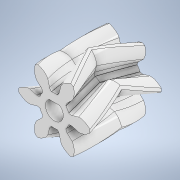
# Autodesk Inventor part: DoubleHelicalDriveGear
Saved by Autodesk Inventor 2020.2 (Build 242310000, 310)
## iProperties
Created: 2019-09-23
Part Number: DoubleHelicalDriveGear
Material: Generic
Document SubType Name: Modeling
Designer: Eric
Density: 1 g/cm^3
Appearance: White
ReferenceDiameter: 15.000 mm
Teeth: 6.000 ul
TipDiameter: 20.000 mm
Author: Eric
Autodesk Inventor part; units mm, degrees
ref_plane "YZ Plane" through (0, 0, 0) normal (1, 0, 0) x (0, 1, 0)
ref_plane "XZ Plane" through (0, 0, 0) normal (0, 1, 0) x (-1, 0, 0)
ref_plane "XY Plane" through (0, 0, 0) normal (0, 0, 1) x (1, 0, 0)
sketch "Sketch1" plane through (0, 0, 0) normal (0, 0, 1) x (1, 0, 0)
  circle A0 centre (0, 0) radius 7.0477
  circle A1 centre (0, 0) radius 7.5
  circle A2 centre (0, 0) radius 10
  circle A3 centre (0, 0) radius 4.375
  line L0 (-14, 0) -> (14, 0) projected
  line L1 (0, 0) -> (6.8335, 1.7241)
  line L2 (7.2444, 1.9411) -> (0, 0)
  line L3 (7.2444, 1.9411) -> (0, 0)
  circle A4 centre (0, 0) radius 7.0477
  dimension "BaseDiameter" = 14.0954
  dimension "RootDiameter" = 8.75
  dimension "ReferenceDiameter" = 15
  dimension "TipDiameter" = 20
  dimension "d26" = 15
  dimension "d30" = 15
  dimension "d48" = 0.7398
  constraints: 6 end point, 4 coincident, 3 centre point, 2 horizontal, 2 point on circle, 1 line through centre, 1 point on line, 20 other
  measures "ReferenceDiameter" diameter of A1
  measures "TipDiameter" diameter of A2
  measures "d26" angle of L0 L2
  measures "d30" angle of L0 L3
  measures "d48" distance from line of L0 point (4.312, 0.74)
extrude "Extrusion3" add sketch "Sketch1" along normal blind 10
sketch "Sketch3" plane through (0, 0, 0) normal (0, 0, 1) x (1, 0, 0)
  circle A0 centre (0, 0) radius 10 projected
  circle A1 centre (0, 0) radius 4.375 projected
  line L0 (0, 0) -> (6.8335, 1.7241) projected
  spline S0 degree 3 poles (4.312, 0.7398) (4.6304, 1.2842) (5.5617, 1.5626) (6.6593, 1.13) (7.1921, 0.9201) (7.7578, 0.5477) (8.2812, 0) knots -0.027536 -0.027536 -0.027536 -0.027536 0.566373 0.566373 0.566373 0.854705 0.854705 0.854705 0.854705 projected
  spline S1 degree 3 poles (6.8335, 1.7241) (6.9431, 1.7526) (7.0448, 1.8131) (7.1455, 1.8759) (7.8344, 2.3054) (8.4145, 3.1058) (8.8099, 4.097) (8.9564, 4.4642) (9.0767, 4.8606) (9.1662, 5.2815) knots 1 1 1 1 1.048198 1.048198 1.048198 1.377882 1.377882 1.377882 1.5 1.5 1.5 1.5 projected
  circle A2 centre (0, 0) radius 10 projected
  circle A3 centre (0, 0) radius 4.275
  line L1 (-0.0245, 0.097) -> (6.8087, 1.821)
  line L2 (-14, 0) -> (14, 0) projected
  arc A4 (4.217, 0.7953) -> (4.2088, 0.7493) centre (4.2755, 0.7611) ccw
  line L3 (-0.0245, -0.097) -> (6.8087, -1.821)
  spline S2 degree 3 poles (4.312, -0.7398) (4.6304, -1.2842) (5.5617, -1.5626) (6.6593, -1.13) (7.1921, -0.9201) (7.7578, -0.5477) (8.2812, 0) knots -0.027536 -0.027536 -0.027536 -0.027536 0.566373 0.566373 0.566373 0.854705 0.854705 0.854705 0.854705 projected
  spline S3 degree 3 poles (6.8335, -1.7241) (6.9431, -1.7526) (7.0448, -1.8131) (7.1455, -1.8759) (7.8344, -2.3054) (8.4145, -3.1058) (8.8099, -4.097) (8.9564, -4.4642) (9.0767, -4.8606) (9.1662, -5.2815) knots 1 1 1 1 1.048198 1.048198 1.048198 1.377882 1.377882 1.377882 1.5 1.5 1.5 1.5 projected
  arc A5 (4.2088, -0.7493) -> (4.217, -0.7953) centre (4.2755, -0.7611) ccw
  spline S4 degree 5 poles (6.8084, 1.8209) (6.92, 1.8489) (7.0177, 1.9142) (7.1157, 1.9709) (7.3162, 2.1084) (7.5003, 2.2658) (7.5937, 2.3536) (7.7795, 2.5454) (7.9485, 2.7523) (8.032, 2.8636) (8.197, 3.1007) (8.3448, 3.349) (8.417, 3.4803) (8.5577, 3.7556) (8.6812, 4.039) (8.7409, 4.1868) (8.8542, 4.4951) (8.9494, 4.8095) (8.9936, 4.9727) (9.0332, 5.137) (9.0684, 5.3023) knots 0 0 0 0 0 0 0.13312 0.13312 0.13312 0.281917 0.281917 0.281917 0.443673 0.443673 0.443673 0.617928 0.617928 0.617928 0.803317 0.803317 0.803317 1 1 1 1 1 1
  spline S5 degree 5 poles (4.217, 0.7953) (4.3335, 0.995) (4.5086, 1.1604) (4.7136, 1.278) (5.2244, 1.4662) (5.7727, 1.4747) (6.0806, 1.434) (6.7834, 1.2483) (7.4202, 0.8925) (7.7605, 0.6506) (8.074, 0.3759) (8.3607, 0.076) knots 0 0 0 0 0 0 0.242405 0.242405 0.242405 0.564814 0.564814 0.564814 1 1 1 1 1 1
  spline S6 degree 5 poles (6.8084, -1.8209) (6.92, -1.8489) (7.0177, -1.9142) (7.1157, -1.9709) (7.3162, -2.1084) (7.5003, -2.2658) (7.5937, -2.3536) (7.7795, -2.5454) (7.9485, -2.7523) (8.032, -2.8636) (8.197, -3.1007) (8.3448, -3.349) (8.417, -3.4803) (8.5577, -3.7556) (8.6812, -4.039) (8.7409, -4.1868) (8.8542, -4.4951) (8.9494, -4.8095) (8.9936, -4.9727) (9.0332, -5.137) (9.0684, -5.3023) knots 0 0 0 0 0 0 0.13312 0.13312 0.13312 0.281917 0.281917 0.281917 0.443673 0.443673 0.443673 0.617928 0.617928 0.617928 0.803317 0.803317 0.803317 1 1 1 1 1 1
  spline S7 degree 5 poles (4.217, -0.7953) (4.3335, -0.995) (4.5086, -1.1604) (4.7136, -1.278) (5.2244, -1.4662) (5.7727, -1.4747) (6.0806, -1.434) (6.7834, -1.2483) (7.4202, -0.8925) (7.7605, -0.6506) (8.074, -0.3759) (8.3607, -0.076) knots 0 0 0 0 0 0 0.242405 0.242405 0.242405 0.564814 0.564814 0.564814 1 1 1 1 1 1
  point P0 (4.9793, 1.3594)
  point P1 (4.9793, -1.3594)
  point P2 (8.8818, -4.595)
  point P3 (8.8818, 4.595)
  point P4 (6.8087, 1.821)
  dimension "d113" = 0.11
  dimension "d114" = 0.11
  dimension "d111" = 0.1
  dimension "d112" = 0.1
  constraints: 8 point on circle, 6 coincident, 4 end point, 3 centre point, 2 point on line, 2 symmetric about line, 2 tangent, 1 parallel, 18 other
  measures "d111" radial gap between concentric circles of A1 A3
  measures "d112" distance between parallel lines of L0 L1
sketch "Sketch11" plane through (0, 0, 10) normal (0, 0, 1) x (1, 0, 0)
  circle A0 centre (0, 0) radius 2.5
  line L0 (-1.5, 2) -> (1.5, 2)
  dimension "d101" = 5
  dimension "d102" = 4.5
  constraints: 2 coincident, 2 end point, 2 point on circle, 1 centre point, 1 horizontal
  measures "d101" diameter of A0
extrude "Extrusion8" cut sketch "Sketch11" against normal through all contours A0 L0 picked at (0.1119, 0.5076)
coil "Coil3" sketch "Sketch3" operation cut axis through (0, 0, -10) along (0, 0, 1) pitch 120 turns 0.083333 hand left contours L2 S0 A1 S5 L0 S1 A0 | A0 S6 L3 S7 A1 S2 L2 | S1 L0 S5 L1 S4 A0 | L2 A1 S0 | S2 A1 L2 | A1 L2 A3 A4 S5 | A1 S7 A5 A3 L2 | L0 S5 L1
pattern_circular "Circular Pattern5" count 6 over 360 about axis through (0, 0, -10) along (0, 0, 1) of "Coil3"
mirror "Mirror4" about plane through (0, 0, 0) normal (0, 0, 1)
equation "\"Module\" = 2.5"
equation "\"PressureAngle\" = 20deg"
equation "\"Teeth\" = 6"
equation "\"TorochoidHeight\" = 0.73979"
equation "\"Clearance\" = 0.1"
body "Solid2"
